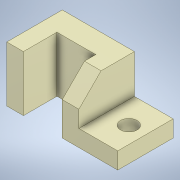
# Autodesk Inventor part: INVENTOR_TUT
Saved by Autodesk Inventor 2021.1 (Build 251245000, 245)
## iProperties
Created: 2021-05-10
Part Number: INVENTOR_TUT
Material: Polypropylene
Document SubType Name: Modeling
Designer: as000166
Density: 0.899 g/cm^3
Appearance: Smooth - Ash
Mass: 239.732 g
Surface Area: 374.755 cm^2
Volume: 266.666 cm^3
Author: as000166
Autodesk Inventor part; units mm, degrees
ref_plane "YZ Plane" through (0, 0, 0) normal (1, 0, 0) x (0, 1, 0)
ref_plane "XZ Plane" through (0, 0, 0) normal (0, 1, 0) x (-1, 0, 0)
ref_plane "XY Plane" through (0, 0, 0) normal (0, 0, 1) x (1, 0, 0)
sketch "Sketch1" plane through (0, 0, 0) normal (0, 0, 1) x (1, 0, 0)
  line L0 (0, 0) -> (0, 63.5)
  line L1 (0, 63.5) -> (19.05, 63.5)
  line L2 (0, 0) -> (63.5, 0)
  line L3 (63.5, 0) -> (63.5, 19.05)
  line L4 (63.5, 19.05) -> (19.05, 19.05)
  line L5 (19.05, 19.05) -> (19.05, 63.5)
  dimension "d3" = 63.5
  dimension "d6" = 19.05
  dimension "d7" = 63.5
  dimension "d8" = 19.05
  dimension "d9" = 44.45
  dimension "d10" = 44.45
  constraints: 12 end point, 2 horizontal, 2 perpendicular, 2 vertical
  measures "d3" distance of L0.start L0.end
  measures "d6" distance of L0.end L1.end
  measures "d7" distance of L0.start L2.end
  measures "d8" distance of L2.end L3.end
  measures "d9" distance of L4.end L1.end
  measures "d10" distance of L3.end L4.end
extrude "Extrusion1" add sketch "Sketch1" along normal blind 63.5
sketch "Sketch2" plane through (0, 63.5, 0) normal (0, 1, 0) x (1, 0, 0)
  line L0 (0, 0) -> (-63.5, 0)
  line L1 (-63.5, 0) -> (-63.5, -63.5)
  line L2 (-63.5, -63.5) -> (-44.45, -63.5)
  line L3 (0, 0) -> (0, -63.5) projected
  line L4 (0, -6.0479) -> (0, -25.0979)
  line L5 (0, -25.0979) -> (-44.45, -25.0979)
  line L6 (-44.45, -25.0979) -> (-44.45, -63.5)
  dimension "d19" = 63.5
  dimension "d20" = 63.5
  dimension "d21" = 19.05
  dimension "d22" = 19.05
  dimension "d23" = 38.4021
  dimension "d24" = 44.45
  constraints: 12 end point, 3 perpendicular, 2 point on line, 1 horizontal, 1 vertical
  measures "d19" distance of L0.start L0.end
  measures "d20" distance of L0.end L1.end
  measures "d21" distance of L1.end L2.end
  measures "d22" distance of L4.start L4.end
  measures "d23" distance of L5.end L2.end
  measures "d24" distance of L4.end L5.end
extrude "Extrusion2" add sketch "Sketch2" against normal blind 63.5
sketch "Sketch3" plane through (19.05, 19.05, 0) normal (0, 1, 0) x (1, 0, 0)
  line L0 (44.45, 0) -> (44.45, -63.5) projected
  line L1 (-82.55, 0) -> (44.45, 0) projected
  circle A0 centre (25.4, -31.75) radius 9.525
  point P0 (-19.05, 0)
  dimension "d29" = 19.05
  constraints: 1 centre point
  measures "d29" diameter of A0
extrude "Extrusion3" cut sketch "Sketch3" along normal blind 63.5 and the other way blind 31.75
sketch "Sketch4" plane through (19.05, 19.05, 0) normal (1, 0, 0) x (0, 0, -1)
  line L0 (-63.5, 44.45) -> (-25.0979, 44.45) projected
  line L1 (-63.5, 44.45) -> (-38.1, 44.45)
  line L2 (-38.1, 44.45) -> (-63.1713, 19.3817)
  line L3 (-63.1713, 19.3817) -> (-63.5, 19.0531)
  line L4 (-63.5, 44.45) -> (-63.5, -19.05) projected
  point P0 (0, -19.05)
  dimension "d34" = 25.4
  constraints: 6 end point, 3 point on line
  measures "d34" distance of L0.start L1.end
extrude "Extrusion4" cut sketch "Sketch4" against normal blind 50.8
body "Solid1"
